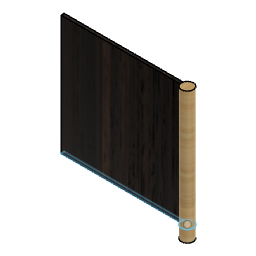
_4 per exterior.0b685afe-bdc7-46a3-a487-12d08d3ee605 (Autodesk Fusion 360 design; units mm, degrees)
Autodesk Fusion 360 part; units mm, degrees
sketch "sketch 329" plane through (0, 0, 0) normal (0, 0, 1) x (1, 0, 0)
  line L0 (-592.1542, 33.8806) -> (-718.1418, 33.8806)
  line L1 (-592.1542, 37.0302) -> (-592.1542, 33.8806)
  line L2 (-718.1418, 37.0302) -> (-592.1542, 37.0302)
  line L3 (-718.1418, 33.8806) -> (-718.1418, 37.0302)
  circle A0 centre (-585.7679, 35.4554) radius 6.35
extrude "Extrude1" add sketch "sketch 329" along normal blind 127 makes body 1 at (-634.15, 33.8806, 84.6667) makes body 2 at (-585.6096, 41.8034, 84.6667)
extrude "Extrude2" add 1 faces at (-584.019, 37.2787, 0) along direction (0, 0, -1) blind 12.7 on bodies 2 bodies 2
